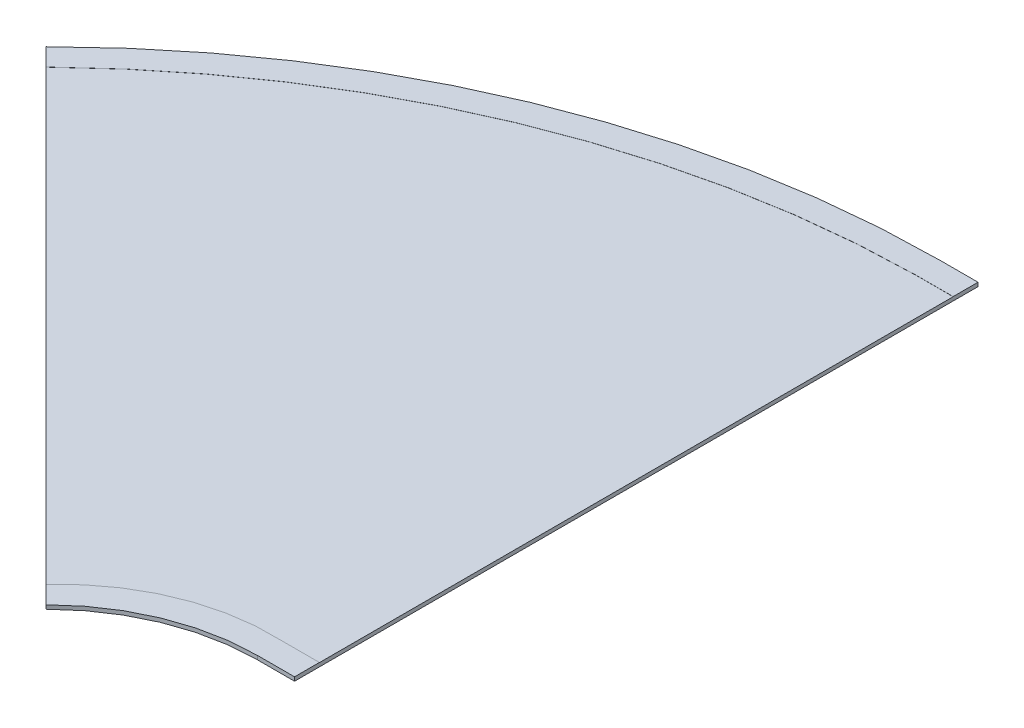
# Autodesk Inventor part: curve_left
Saved by Autodesk Inventor 2021 (Build 250183000, 183)
## iProperties
Created: 2021-01-02
Part Number: curve_left
Material: Generic
Document SubType Name: Modeling
Designer: Tomasz
Density: 1 g/cm^3
Appearance: Default
Author: Tomasz
Autodesk Inventor part; units mm, degrees
ref_plane "YZ Plane" through (0, 0, 0) normal (1, 0, 0) x (0, 1, 0)
ref_plane "XZ Plane" through (0, 0, 0) normal (0, 1, 0) x (-1, 0, 0)
ref_plane "XY Plane" through (0, 0, 0) normal (0, 0, 1) x (1, 0, 0)
sketch "Sketch1" plane through (0, 0, 0) normal (0, 1, 0) x (-1, 0, 0)
  line L0 (30, 275) -> (0, 275)
  line L1 (0, 275) -> (0, -275)
  line L2 (0, -275) -> (30, -275)
  line L3 (30, -275) -> (30, 275)
  arc A0 (30, -275) -> (539.12, -64.1138) centre (30, 445) ccw
  arc A1 (30, 275) -> (150.2089, 324.7926) centre (30, 445) ccw
  line L4 (150.2089, 324.7926) -> (539.12, -64.1138)
  line L5 (0, 255) -> (30, 255)
  line L6 (0, -255) -> (30, -255)
  arc A2 (30, 255) -> (164.3511, 310.6505) centre (38.3697, 424.7938) ccw
  arc A3 (30, -255) -> (524.9778, -49.9717) centre (21.7353, 464.9526) ccw
  point P0 (0, 0)
  point P1 (0, 0)
  point P2 (344.6644, 130.3394)
  dimension "d0" = 30
  dimension "d1" = 550
  dimension "d2" = 720
  dimension "d3" = 170
  dimension "d4" = 550
  dimension "d5" = 539.12
  dimension "d10" = 20
  dimension "d11" = 20
  dimension "d12" = 20
  dimension "d13" = 20
  dimension "d16" = 130.3394
  dimension "d17" = 344.6644
  dimension "d19" = 170
  dimension "d20" = 720
  constraints: 14 end point, 8 point on circle, 6 point on line, 4 centre point, 3 parallel, 2 midpoint, 2 perpendicular, 1 coincident, 1 concentric, 1 horizontal
  measures "d0" distance of L2.end L1.end
  measures "d1" distance of L1.end L0.end
  measures "d2" radius of A0
  measures "d3" radius of A1
  measures "d4" distance of L4.start L4.end
  measures "d5" distance from line of L4.end L1
  measures "d10" distance of L4.start A2.end
  measures "d11" distance of L0.end L5.start
  measures "d12" distance of L1.end L6.start
  measures "d13" distance of L4.end A3.end
  measures "d16" vertical distance of point (0, 0) point (344.664, 130.339)
  measures "d17" horizontal distance of point (0, 0) point (344.664, 130.339)
  measures "d19" radius of A2
  measures "d20" radius of A3
extrude "Extrusion1" add sketch "Sketch1" along normal blind 3
extrude "Extrusion2" add sketch "Sketch1" along normal blind 3.1 contours L3 L5 L1 L0 | A1 L4 A2 L3 | A3 L4 A0 L3 | L3 L2 L1 L6
equation "\"d1\" = d4"
equation "\"d4\" = track_width"
equation "\"d10\" = curb_width"
equation "\"d11\" = curb_width"
equation "\"d12\" = curb_width"
equation "\"d13\" = curb_width"
equation "\"d19\" = d3"
equation "\"d20\" = d2"
equation "\"d6\" = track_height"
equation "\"d14\" = track_height + curb_height"
equation "\"track_width\" = 550"
equation "\"curb_width\" = 20"
equation "\"track_height\" = 3"
equation "\"curb_height\" = 0.1"
body "Solid1"
